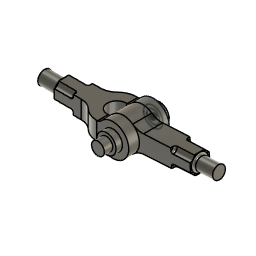
Knuckle Joint_ (Autodesk Fusion 360 design; units mm, degrees)
Autodesk Fusion 360 part; units mm, degrees
sketch "Sketch1" plane through (0, 0, 0) normal (0, 0, 1) x (1, 0, 0) in component "fork"
  line L0 (101.25, 47.5) -> (25.75, 47.5)
  line L1 (25.75, -47.5) -> (101.25, -47.5)
  line L2 (25.7534, 22.5) -> (101.25, 22.5)
  line L3 (101.25, -22.5) -> (25.7534, -22.5)
  line L4 (-16.083, 22.5) -> (-99.1929, 22.5)
  line L5 (-99.1929, 22.5) -> (-99.1929, -22.5)
  line L6 (-99.1929, -22.5) -> (-16.083, -22.5)
  arc A0 (25.7534, 22.5) -> (25.7534, -22.5) centre (25.75, 0) ccw
  line L7 (101.25, -47.5) -> (101.25, -22.5)
  line L8 (101.25, 22.5) -> (101.25, 47.5)
  arc A1 (25.75, 47.5) -> (25.75, -47.5) centre (25.75, 0) ccw
  dimension "d4" = 45
  dimension "d7" = 45
  dimension "d8" = 45
  constraint horizontal L0
  constraint parallel L0 L1
  constraint horizontal L2
  constraint horizontal L3
  constraint horizontal L4
  constraint perpendicular L4 L5
  constraint parallel L4 L6
  constraint collinear L7 L8
  measures "d4" diameter of A0
  measures "d7" distance of L2.start L3.end
  measures "d8" distance of L4.end L5.end
extrude "Extrude1" add sketch "Sketch1" along normal mid plane 80 makes body 1 in component "fork"
sketch "Sketch2" plane through (0, -47.5, 0) normal (0, -1, 0) x (1, 0, 0) in component "fork"
  line L0 (101.25, -40) -> (101.25, 40)
  line L1 (101.25, 40) -> (25.75, 40)
  line L2 (25.75, 40) -> (25.75, -40)
  line L3 (25.75, -40) -> (101.25, -40)
  circle A0 centre (63.75, 0) radius 15
  circle A1 centre (63.75, 0) radius 37.5
  line L4 (32.6815, 21) -> (-111.3185, 21)
  line L5 (-111.3185, 21) -> (-111.3185, -21)
  line L6 (-111.3185, -21) -> (32.6815, -21)
  line L7 (32.6815, -21) -> (32.6815, 21)
  dimension "d11" = 30
  dimension "d12" = 75
  dimension "d13" = 42
  dimension "d14" = 144
  constraint concentric A0 A1
  constraint tangent L0 A1
  constraint horizontal L4
  constraint vertical L5
  constraint horizontal L6
  constraint vertical L7
  constraint coincident A1 L4.start
  constraint coincident A1 L6.end
  measures "d11" diameter of A0
  measures "d12" diameter of A1
  measures "d13" distance of L4.start L6.end
  measures "d14" distance of L4.start L4.end
extrude "Extrude2" cut sketch "Sketch2" against normal blind 120 contours A1 L7 | A1 L7 | L2 A1 L4 L6 | L2 L4 L5 L6 keep common part bodies 1 in component "fork"
fillet "Fillet1" radius 10 4 edges at (32.6815, 35, 21) (32.6815, -35, 21) (32.6815, -35, -21) (32.6815, 35, -21) on bodies 1 in component "fork"
fillet "Fillet2" radius 40 2 edges at (-16.083, -22.5, 0) (-16.083, 22.5, 0) on bodies 1 in component "fork"
sketch "Sketch3" plane through (-99.1929, 0, 0) normal (-1, 0, 0) x (0, -1, 0) in component "fork"
  line L0 (-22.5, -21) -> (22.5, -21)
  line L1 (22.5, -21) -> (22.5, 21)
  line L2 (22.5, 21) -> (-22.5, 21)
  line L3 (-22.5, 21) -> (-22.5, -21)
  circle A0 centre (22.5, 21) radius 10.5
  circle A1 centre (-22.5, 21) radius 10.5
  circle A2 centre (-22.5, -21) radius 10.5
  circle A3 centre (22.5, -21) radius 10.5
  dimension "d21" = 21
  dimension "d22" = 21
  dimension "d23" = 21
  dimension "d24" = 21
  constraint coincident L1.end L2.start
  constraint coincident L2.end L3.start
  constraint coincident L0.start L3.end
  constraint coincident L0.end L1.start
  measures "d21" diameter of A0
  measures "d22" diameter of A1
  measures "d23" diameter of A2
  measures "d24" diameter of A3
extrude "Extrude3" cut sketch "Sketch3" against normal blind 45 contours L0 L3 A2 | L0 L1 A3 | L2 L3 A1 | L1 L2 A0 picked at (-15.5356, -20.5019) picked at (18.3157, -15.4105) picked at (-15.5356, 20.5019) picked at (15.5356, 20.5019) bodies 1 in component "fork"
fillet "Fillet3" radius 5 4 edges at (-54.1929, 15.0754, -13.5754) (-54.1929, -15.0754, -13.5754) (-54.1929, 15.0754, 13.5754) (-54.1929, -15.0754, 13.5754) on bodies 1 in component "fork"
sketch "Sketch4" plane through (-99.1929, 0, 0) normal (-1, 0, 0) x (0, -1, 0) in component "fork"
  arc A0 (12, 21) -> (22.5, 10.5) centre (22.5, 21) ccw
  line L0 (12, 21) -> (-12, 21)
  arc A1 (-22.5, 10.5) -> (-12, 21) centre (-22.5, 21) ccw
  line L1 (-22.5, 10.5) -> (-22.5, -10.5)
  arc A2 (-12, -21) -> (-22.5, -10.5) centre (-22.5, -21) ccw
  line L2 (-12, -21) -> (12, -21)
  arc A3 (22.5, -10.5) -> (12, -21) centre (22.5, -21) ccw
  line L3 (22.5, -10.5) -> (22.5, 10.5)
  circle A4 centre (0, 0) radius 16
  dimension "d29" = 32
  constraint coincident A4.centre origin
  measures "d29" diameter of A4
extrude "Extrude4" add sketch "Sketch4" along normal blind 45 contours A4 bodies 1 in component "fork"
fillet "Fillet4" radius 5 1 edges at (-99.1929, 14.9172, 5.7858) on bodies 1 in component "fork"
sketch "Sketch1 (2)" plane through (0, 0, 0) normal (0, 0, 1) x (1, 0, 0) in component "eye rod"
  line L0 (-99.1929, 22.5) -> (-99.1929, 21)
  line L1 (-99.1929, -21) -> (-99.1929, -22.5)
  line L2 (-144.1929, 16) -> (-144.1929, -16)
  line L3 (-54.1929, -22.5) -> (-59.1929, -22.5)
  line L4 (-59.1929, 22.5) -> (-54.1929, 22.5)
  line L5 (-99.1929, -22.5) -> (-59.1929, -22.5)
  line L6 (-59.1929, 22.5) -> (-99.1929, 22.5)
  line L7 (-54.1929, 22.5) -> (-35.4872, 22.5)
  arc A0 (-35.4872, 22.5) -> (-7.4931, 33.9286) centre (-35.4872, 62.5) ccw
  arc A1 (-7.4931, -33.9286) -> (-35.4872, -22.5) centre (-35.4872, -62.5) ccw
  arc A2 (-7.4931, -33.9286) -> (25.75, -47.5) centre (25.75, 0) ccw
  line L8 (35.3372, 22.5) -> (27.7604, 22.5)
  line L9 (27.7604, 47.5) -> (35.3372, 47.5)
  arc A3 (25.75, 47.5) -> (-7.4931, 33.9286) centre (25.75, 0) ccw
  line L10 (25.75, 47.5) -> (27.7604, 47.5)
  line L11 (27.7604, 22.5) -> (25.7534, 22.5)
  arc A4 (25.7534, 22.5) -> (25.7534, -22.5) centre (25.75, 0) ccw
  line L12 (25.7534, -22.5) -> (27.7604, -22.5)
  line L13 (27.7604, -47.5) -> (25.75, -47.5)
  line L14 (-35.4872, -22.5) -> (-54.1929, -22.5)
  line L15 (27.7604, -22.5) -> (35.3372, -22.5)
  line L16 (35.3372, -47.5) -> (27.7604, -47.5)
  line L17 (35.3372, -22.5) -> (101.25, -22.5)
  line L18 (101.25, -47.5) -> (35.3372, -47.5)
  line L19 (35.3372, 47.5) -> (101.25, 47.5)
  line L20 (101.25, 22.5) -> (35.3372, 22.5)
  arc A5 (-104.1929, 16) -> (-99.1929, 21) centre (-104.1929, 21) ccw
  arc A6 (-99.1929, -21) -> (-104.1929, -16) centre (-104.1929, -21) ccw
  line L21 (-104.1929, 16) -> (-144.1929, 16)
  line L22 (-104.1929, -16) -> (-144.1929, -16)
  line L23 (101.25, -47.5) -> (101.25, -22.5)
  line L24 (101.25, 22.5) -> (101.25, 47.5)
  line L25 (26.25, 22.5) -> (221.25, 22.5)
  line L26 (221.25, 22.5) -> (221.25, -22.5)
  line L27 (221.25, -22.5) -> (26.25, -22.5)
  line L28 (26.25, -22.5) -> (26.25, 22.5)
  dimension "d34" = 75
  dimension "d35" = 195
  constraint horizontal L25
  constraint vertical L26
  constraint horizontal L27
  constraint vertical L28
  constraint coincident L17 L26.end
  constraint coincident L20 L25.start
  measures "d34" distance of L24 L28
  measures "d35" distance of L26 L28
extrude "Extrude1'" add sketch "Sketch1 (2)" along normal mid plane 80 separate body contours L8 L11 L12 L15 L17 L20 L25 L26 L27 L28 makes body 2 in component "eye rod"
sketch "Sketch2 (2)" plane through (0, -22.5, 0) normal (0, -1, 0) x (1, 0, 0) in component "eye rod"
  line L0 (221.25, -40) -> (221.25, 40)
  line L1 (221.25, 40) -> (26.25, 40)
  line L2 (26.25, 40) -> (26.25, -40)
  line L3 (26.25, -40) -> (221.25, -40)
  circle A0 centre (63.7469, 0) radius 37.5
  circle A1 centre (63.7469, 0) radius 15
  line L4 (95.0847, -20.5959) -> (1091.9409, -20.5959)
  line L5 (1091.9409, -20.5959) -> (1091.9409, 20.5959)
  line L6 (1091.9409, 20.5959) -> (95.0847, 20.5959)
  line L7 (95.0847, 20.5959) -> (95.0847, -20.5959)
  dimension "d38" = 75
  dimension "d39" = 30
  constraint concentric A0 A1
  constraint horizontal L4
  constraint vertical L5
  constraint horizontal L6
  constraint vertical L7
  constraint coincident A0 L4.start
  constraint coincident A0 L6.end
  measures "d38" diameter of A0
  measures "d39" diameter of A1
extrude "Extrude2'" cut sketch "Sketch2 (2)" against normal blind 70 contours L0 A0 L4 L6 | A0 L7 | L2 A0 L7 keep common part bodies 2 in component "eye rod"
fillet "Fillet1'" radius 40 2 edges at (95.0847, 0, 20.5959) (95.0847, 0, -20.5959) on bodies 2 in component "eye rod"
sketch "Sketch3 (2)" plane through (221.25, 0, 0) normal (1, 0, 0) x (0, 1, 0) in component "eye rod"
  line L0 (-22.5, -20.5959) -> (22.5, -20.5959)
  line L1 (22.5, -20.5959) -> (22.5, 20.5959)
  line L2 (22.5, 20.5959) -> (-22.5, 20.5959)
  line L3 (-22.5, 20.5959) -> (-22.5, -20.5959)
  circle A0 centre (22.5, 20.5959) radius 10.5
  circle A1 centre (-22.5, 20.5959) radius 10.5
  circle A2 centre (-22.5, -20.5959) radius 10.5
  circle A3 centre (22.5, -20.5959) radius 10.5
  dimension "d46" = 21
  dimension "d47" = 21
  dimension "d48" = 21
  dimension "d49" = 21
  constraint coincident L1.end L2.start
  constraint coincident L2.end L3.start
  constraint coincident L0.start L3.end
  constraint coincident L0.end L1.start
  measures "d46" diameter of A0
  measures "d47" diameter of A1
  measures "d48" diameter of A2
  measures "d49" diameter of A3
extrude "Extrude3'" cut sketch "Sketch3 (2)" against normal blind 45 contours L0 L3 A2 | L0 L1 A3 | L2 L3 A1 | L1 L2 A0 picked at (-15.5356, -20.0978) picked at (16.9105, -16.4116) picked at (-15.5356, 20.0978) picked at (15.5356, 20.0978) bodies 2 in component "eye rod"
fillet "Fillet2'" radius 5 4 edges at (176.25, -15.0754, -13.1713) (176.25, 15.0754, -13.1713) (176.25, 15.0754, 13.1713) (176.25, -15.0754, 13.1713) on bodies 2 in component "eye rod"
cylinder "CylinderPrimitive1" add diameter 30 height 45 placed x (0, 0, -1) y (0, 1, 0) z (1, 0, 0) at (221.25, 0, 0) bodies 2 in component "eye rod"
fillet "Fillet3'" radius 5 1 edges at (221.25, 5.4242, 13.9849) on bodies 2 in component "eye rod"
sketch "Sketch1 (3)" plane through (0, 47.5, 0) normal (0, 1, 0) x (-1, 0, 0) in component "pin"
  circle A0 centre (-63.75, 0) radius 15
  line L0 (-27.7604, -21) -> (-25.75, -21)
  line L1 (-25.75, -21) -> (-25.75, 21)
  line L2 (-25.75, 21) -> (-27.7604, 21)
  arc A1 (-35.3372, 24.4737) -> (-27.7604, 21) centre (-27.7604, 31) ccw
  arc A2 (-35.3372, 24.4737) -> (-35.3372, -24.4737) centre (-63.75, 0) ccw
  arc A3 (-27.7604, -21) -> (-35.3372, -24.4737) centre (-27.7604, -31) ccw
  circle A4 centre (-63.75, 0) radius 15
  circle A5 centre (-63.75, 0) radius 22.5
  dimension "d59" = 30
  dimension "d60" = 45
  constraint concentric A0 A4
  constraint concentric A4 A5
  measures "d59" diameter of A4
  measures "d60" diameter of A5
extrude "Extrude1''" add sketch "Sketch1 (3)" against normal blind 130 separate body contours A0 A4 makes body 3 in component "pin"
extrude "Extrude2''" add sketch "Sketch1 (3)" along normal blind 15 contours A0 A4 | A5 bodies 3 in component "pin"
sketch "Sketch2 (3)" plane through (0, -47.5, 0) normal (0, -1, 0) x (1, 0, 0) in component "pin"
  arc A0 (35.3372, -24.4737) -> (27.7604, -21) centre (27.7604, -31) ccw
  arc A1 (35.3372, -24.4737) -> (35.3372, 24.4737) centre (63.75, 0) ccw
  arc A2 (27.7604, 21) -> (35.3372, 24.4737) centre (27.7604, 31) ccw
  line L0 (27.7604, 21) -> (25.75, 21)
  line L1 (25.75, 21) -> (25.75, -21)
  line L2 (25.75, -21) -> (27.7604, -21)
  circle A3 centre (63.75, 0) radius 15
  circle A4 centre (63.75, 0) radius 22.5
  dimension "d65" = 45
  constraint concentric A1 A4
  measures "d65" diameter of A4
extrude "Extrude3''" add sketch "Sketch2 (3)" along normal blind 15 contours A4 bodies 3 in component "pin"
component "fork" placed x (1, 0, 0) y (0, 1, 0) z (0, 0, 1) at (0, 0, 0)
component "eye rod" placed x (1, 0, 0) y (0, 1, 0) z (0, 0, 1) at (0.0031, 0, 0)
component "pin" placed x (1, 0, 0) y (0, 1, 0) z (0, 0, 1) at (0, 0, 0)
